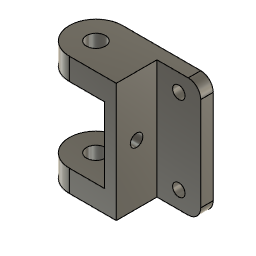
NCV-10 v2 (Autodesk Fusion 360 design; units mm, degrees)
Autodesk Fusion 360 part; units mm, degrees
sketch "Sketch1" plane through (0, 0, 0) normal (0, 0, 1) x (1, 0, 0)
  line L0 (0, 0) -> (-30, 0)
  line L1 (-30, -34) -> (0, -34)
  line L2 (0, -34) -> (0, 0)
  line L3 (0, 0) -> (28, 0)
  line L4 (28, 0) -> (28, -8)
  line L5 (28, -8) -> (0, -8)
  line L6 (0, -8) -> (0, 0)
  arc A0 (-30, 0) -> (-30, -34) centre (-30, -17) ccw
  circle A1 centre (-30, -17) radius 6
  line L7 (-7.5, 0) -> (-7.5, -34)
  dimension "d2" = 28
  dimension "d3" = 8
  dimension "d4" = 34
  dimension "d5" = 34
  dimension "d6" = 17
  dimension "d7" = 12
  dimension "d8" = 30
  dimension "d9" = 7.5
  constraint horizontal L0
  constraint horizontal L1
  constraint vertical L2
  constraint coincident L0.start L2.end
  constraint horizontal L3
  constraint vertical L4
  constraint horizontal L5
  constraint vertical L6
  constraint concentric A0 A1
  constraint coincident L0 L7.start
  constraint coincident L1 L7.end
  constraint vertical L7
  measures "d2" distance of L0.start L4
  measures "d3" distance of L0.start L5
  measures "d4" distance of L0.start L1
  measures "d5" diameter of A0
  measures "d6" vertical distance of L0.start A0.centre
  measures "d7" diameter of A1
  measures "d8" horizontal distance of L0.start A0.centre
  measures "d9" distance of L0.start L7
sketch "Sketch2" plane through (0, 0, 0) normal (0, 1, 0) x (1, 0, 0)
  circle A0 centre (14, -27) radius 4
  line L0 (20, -38) -> (28, -38)
  line L1 (28, -38) -> (28, -30)
  arc A1 (20, -38) -> (28, -30) centre (20, -30) ccw
  dimension "d18" = 8
  dimension "d19" = 27
  dimension "d20" = 14
  dimension "d29" = 16
  dimension "d30" = 38
  dimension "d31" = 28
  constraint horizontal L0
  constraint vertical L1
  constraint tangent L0 A1
  constraint tangent L1 A1
  measures "d18" diameter of A0
  measures "d19" vertical distance of origin A0.centre
  measures "d20" horizontal distance of origin A0.centre
  measures "d30" vertical distance of origin L0.end
  measures "d31" horizontal distance of origin L0.end
sketch "Sketch3" plane through (0, 0, 0) normal (1, 0, 0) x (0, 1, 0)
  circle A0 centre (-21, 0) radius 4
  line L0 (0, 0) -> (-21, 0) construction
  dimension "d22" = 8
  dimension "d23" = 21
  constraint coincident L0.start origin
  constraint coincident A0.centre L0.end
  constraint horizontal L0
  measures "d22" diameter of A0
  measures "d23" distance of A0.centre L0.start
extrude "Extrude1" add sketch "Sketch1" along normal blind 38 and the other way blind 38
extrude "Extrude2" cut sketch "Sketch1" along normal blind 24 and the other way blind 24 contours L0 L1 A0 L7
extrude "Extrude3" cut sketch "Sketch2" against normal through all
extrude "Extrude4" cut sketch "Sketch3" against normal through all
mirror "Mirror1" about plane through (0, 0, 0) normal (0, 0, 1) of "Extrude3"
equation "d4 = ( 17 * 2 ) * 1 mm"
equation "d5 = ( 17 * 2 ) * 1 mm"
equation "d10 = ( 76 / 2 ) * 1 mm"
equation "d12 = ( 76 / 2 ) * 1 mm"
equation "d14 = ( 76 / 2 ) * 1 mm - 14 mm"
equation "d16 = ( 76 / 2 ) * 1 mm - 14 mm"
equation "d19 = ( 76 / 2 ) * 1 mm - 11 mm"
equation "d23 = ( 17 * 2 ) * 1 mm - 13 mm"
equation "d30 = ( 76 / 2 ) * 1 mm"
